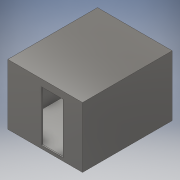
# Autodesk Inventor part: Room
Saved by Autodesk Inventor 2019 (Build 230136000, 136)
## iProperties
Created: 2018-07-10
Part Number: Room
Material: Generic
Document SubType Name: Modeling
Designer: User
Density: 1 g/cm^3
Appearance: Galvanized
Mass: 2.29346e+06 g
Surface Area: 1.09602e+06 cm^2
Volume: 2.29346e+06 cm^3
Author: User
Autodesk Inventor part; units mm, degrees
ref_plane "YZ Plane" through (0, 0, 0) normal (1, 0, 0) x (0, 1, 0)
ref_plane "XZ Plane" through (0, 0, 0) normal (0, 1, 0) x (-1, 0, 0)
ref_plane "XY Plane" through (0, 0, 0) normal (0, 0, 1) x (1, 0, 0)
sketch "Sketch1" plane through (0, 0, 0) normal (0, 1, 0) x (-1, 0, 0)
  line L0 (1524, 1828.8) -> (-1524, 1828.8)
  line L1 (-1524, 1828.8) -> (-1524, -1828.8)
  line L2 (-1524, -1828.8) -> (1524, -1828.8)
  line L3 (1524, -1828.8) -> (1524, 1828.8)
  line L4 (1524, 1828.8) -> (-1524, -1828.8) construction
  line L5 (-1524, 1828.8) -> (1524, -1828.8) construction
  line L6 (-1561.0417, 1873.25) -> (1561.0417, 1873.25)
  line L7 (1561.0417, 1873.25) -> (1561.0417, -1873.25)
  line L8 (1561.0417, -1873.25) -> (-1561.0417, -1873.25)
  line L9 (-1561.0417, -1873.25) -> (-1561.0417, 1873.25)
  line L10 (-1561.0417, 1873.25) -> (1561.0417, -1873.25) construction
  line L11 (1561.0417, 1873.25) -> (-1561.0417, -1873.25) construction
  point P0 (0, 0)
  dimension "d8" = 3048
  dimension "d9" = 3657.6
  dimension "d10" = 44.45
  constraints: 24 end point, 4 midpoint, 4 parallel, 2 horizontal, 2 perpendicular, 1 collinear
  measures "d8" distance of L1.end L2.end
  measures "d9" distance of L2.end L0.start
  measures "d10" distance between parallel lines of L6 L0
extrude "sides" add sketch "Sketch1" along normal mid plane 2438.4
sketch "Sketch2" plane through (0, 1219.2, 0) normal (0, 1, 0) x (1, 0, 0)
  line L0 (1561.0417, 1873.25) -> (-1561.0417, 1873.25) projected
  line L1 (-1561.0417, 1873.25) -> (-1561.0417, -1873.25) projected
  line L2 (1561.0417, -1873.25) -> (1561.0417, 1873.25) projected
  line L3 (-1561.0417, -1873.25) -> (1561.0417, -1873.25) projected
  point P0 (0, 0)
extrude "roof" add sketch "Sketch2" along normal blind 44.45
mirror "floor" about plane through (0, 0, 0) normal (0, 1, 0) of "roof"
sketch "Sketch3" plane through (-1561.0417, 1263.65, 1873.25) normal (0, 0, 1) x (1, 0, 0)
  line L0 (1414.9917, -2393.95) -> (2310.3417, -2393.95)
  line L1 (2310.3417, -2393.95) -> (2310.3417, -285.75)
  line L2 (2310.3417, -285.75) -> (1414.9917, -285.75)
  line L3 (1414.9917, -285.75) -> (1414.9917, -2393.95)
  line L4 (1414.9917, -2393.95) -> (2310.3417, -285.75) construction
  line L5 (2310.3417, -2393.95) -> (1414.9917, -285.75) construction
  line L6 (0, 0) -> (0, -2527.3) projected
  line L7 (0, -2527.3) -> (3122.0833, -2527.3) projected
  line L8 (3122.0833, -2527.3) -> (3122.0833, 0) projected
  line L9 (37.0417, -2482.85) -> (3085.0417, -2482.85) projected
  line L10 (3085.0417, -2482.85) -> (3085.0417, -44.45) projected
  line L11 (3122.0833, -2527.3) -> (3122.0833, 0) projected
  line L12 (0, 0) -> (3122.0833, 0) projected
  line L13 (0, 0) -> (0, -2527.3) projected
  line L14 (0, -2527.3) -> (3122.0833, -2527.3) projected
  point P0 (1561.0417, -1263.65)
  point P1 (1862.6667, -1339.85)
  dimension "d19" = 895.35
  dimension "d20" = 2108.2
  dimension "d22" = 88.9
  dimension "d23" = 774.7
  constraints: 12 end point, 2 midpoint, 2 parallel, 1 horizontal, 1 perpendicular
  measures "d19" distance of L1.end L2.end
  measures "d20" distance of L0.end L1.end
  measures "d22" distance between parallel lines of L9 L0
  measures "d23" distance between parallel lines of L10 L1
extrude "door" cut sketch "Sketch3" against normal up to next contours L3 L2 L1 L0
sketch "Sketch6" plane through (1524, 1219.2, 1828.8) normal (0, 0, -1) x (-1, 0, 0)
  circle A0 centre (2851.15, -2317.75) radius 19.05
  line L0 (3048, -2438.4) -> (0, -2438.4) projected
  line L1 (3048, 0) -> (3048, -2438.4) projected
  point P0 (1524, -1219.2)
  dimension "d24" = 38.1
  dimension "d25" = 120.65
  dimension "d26" = 196.85
  constraints: 1 centre point
  measures "d24" diameter of A0
  measures "d25" distance from line of L0 A0.centre
  measures "d26" distance from line of L1 A0.centre
extrude "Extrusion6" add sketch "Sketch6" along normal blind 63.5
sketch "Sketch8" plane through (0, 1219.2, 0) normal (0, -1, 0) x (1, 0, 0)
  line L0 (863.6, 1371.6) -> (1117.6, 1371.6)
  line L1 (1117.6, 1371.6) -> (1117.6, 1117.6)
  line L2 (1117.6, 1117.6) -> (863.6, 1117.6)
  line L3 (863.6, 1117.6) -> (863.6, 1371.6)
  line L4 (863.6, 1371.6) -> (1117.6, 1117.6) construction
  line L5 (1117.6, 1371.6) -> (863.6, 1117.6) construction
  line L6 (-1092.2, -1397) -> (-838.2, -1397)
  line L7 (-838.2, -1397) -> (-838.2, -1143)
  line L8 (-838.2, -1143) -> (-1092.2, -1143)
  line L9 (-1092.2, -1143) -> (-1092.2, -1397)
  line L10 (-1092.2, -1397) -> (-838.2, -1143) construction
  line L11 (-838.2, -1397) -> (-1092.2, -1143) construction
  line L12 (1524, -1828.8) -> (1524, 1828.8) projected
  line L13 (1524, 1828.8) -> (-1524, 1828.8) projected
  line L14 (-1524, -1828.8) -> (1524, -1828.8) projected
  line L15 (-1524, 1828.8) -> (-1524, -1828.8) projected
  point P0 (0, 0)
  point P1 (990.6, 1244.6)
  point P2 (-965.2, -1270)
  dimension "d29" = 254
  dimension "d30" = 406.4
  dimension "d31" = 457.2
  dimension "d32" = 431.8
  dimension "d33" = 431.8
  constraints: 24 end point, 4 midpoint, 4 parallel, 3 equal length, 2 horizontal, 2 perpendicular
  measures "d29" distance of L0.start L0.end
  measures "d30" distance between parallel lines of L12 L1
  measures "d31" distance between parallel lines of L13 L0
  measures "d32" distance between parallel lines of L14 L6
  measures "d33" distance between parallel lines of L15 L9
extrude "Extrusion7" [suppressed]
sketch "Sketch9" plane through (0, 1263.65, 0) normal (0, 1, 0) x (1, 0, 0)
  line L0 (1561.0417, 1873.25) -> (-1561.0417, 1873.25) projected
  line L1 (-1561.0417, 1873.25) -> (-1561.0417, -1873.25) projected
  line L2 (-1561.0417, -1873.25) -> (1561.0417, -1873.25) projected
  line L3 (1561.0417, -1873.25) -> (1561.0417, 1873.25) projected
  line L4 (1162.05, -1073.15) -> (819.15, -1073.15)
  line L5 (819.15, -1073.15) -> (819.15, -1416.05)
  line L6 (819.15, -1416.05) -> (1162.05, -1416.05)
  line L7 (1162.05, -1416.05) -> (1162.05, -1073.15)
  line L8 (1162.05, -1073.15) -> (819.15, -1416.05) construction
  line L9 (819.15, -1073.15) -> (1162.05, -1416.05) construction
  line L10 (-793.75, 1441.45) -> (-1136.65, 1441.45)
  line L11 (-1136.65, 1441.45) -> (-1136.65, 1098.55)
  line L12 (-1136.65, 1098.55) -> (-793.75, 1098.55)
  line L13 (-793.75, 1098.55) -> (-793.75, 1441.45)
  line L14 (-793.75, 1441.45) -> (-1136.65, 1098.55) construction
  line L15 (-1136.65, 1441.45) -> (-793.75, 1098.55) construction
  line L16 (990.6, -1244.6) -> (1117.6, -1244.6)
  line L17 (1117.6, -1117.6) -> (1117.6, -1371.6) projected
  line L18 (990.6, -1244.6) -> (990.6, -1371.6)
  line L19 (-965.2, 1270) -> (-838.2, 1270)
  line L20 (-965.2, 1270) -> (-965.2, 1143)
  point P0 (0, 0)
  constraints: 32 end point, 5 midpoint, 4 parallel, 3 equal length, 2 horizontal, 2 perpendicular
extrude "Extrusion8" [suppressed]
equation "\"d8\" = roomWidth"
equation "\"d9\" = roomDepth"
equation "\"d10\" = wallThick"
equation "\"d11\" = roomHeight"
equation "\"d13\" = wallThick"
equation "\"d19\" = doorWidth"
equation "\"d20\" = doorHeight"
equation "\"d22\" = doorY"
equation "\"d23\" = doorX"
equation "\"d15\" = wallThick"
equation "\"wallThick\" = 44.45"
equation "\"roomWidth\" = 3048"
equation "\"roomDepth\" = 3657.6"
equation "\"roomHeight\" = 2438.4"
equation "\"doorWidth\" = 895.35"
equation "\"doorHeight\" = 2108.2"
equation "\"doorX\" = 774.7"
equation "\"doorY\" = 88.9"
equation "\"doorThick\" = 57.15"
equation "\"doorLip\" = 76.2"
equation "\"tubeR\" = 304.8"
equation "\"tubeTurnR\" = 76.2"
equation "\"tubeD\" = 19.05"
body "Solid3"
